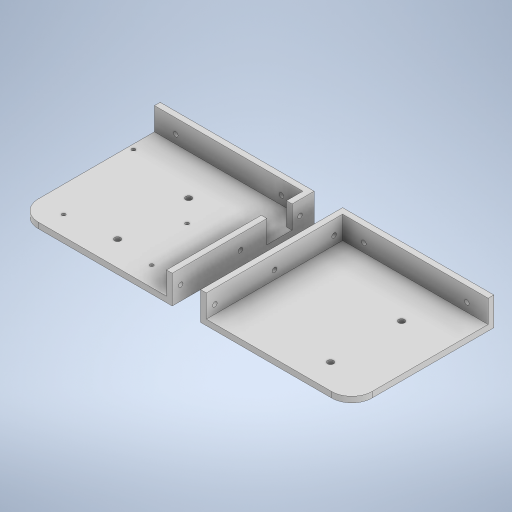
# Autodesk Inventor part: electronics mount
Saved by Autodesk Inventor 2023.1 (Build 271208000, 208)
## iProperties
Created: 2022-11-03
Part Number: electronics mount
Material: Generic
Document SubType Name: Modeling
Designer: nicol
Density: 1 g/cm^3
Appearance: Default
Author: nicol
Autodesk Inventor part; units mm, degrees
ref_plane "YZ Plane" through (0, 0, 0) normal (1, 0, 0) x (0, 1, 0)
ref_plane "XZ Plane" through (0, 0, 0) normal (0, 1, 0) x (-1, 0, 0)
ref_plane "XY Plane" through (0, 0, 0) normal (0, 0, 1) x (1, 0, 0)
sketch "Sketch1" plane through (0, 0, 0) normal (0, 1, 0) x (-1, 0, 0)
  line L0 (108.5, -115) -> (0, -115) construction
  line L1 (0, -115) -> (0, 169.9168) construction
  line L2 (88.5, 0) -> (-126.5, 0) construction
  line L3 (-126.5, 0) -> (-126.5, -115) construction
  line L4 (-126.5, -115) -> (88.5, -115) construction
  line L5 (88.5, -115) -> (88.5, 0) construction
  line L6 (108.5, -15) -> (0, -15)
  line L7 (0, -15) -> (0, -115)
  line L8 (0, -115) -> (108.5, -115)
  line L9 (108.5, -115) -> (108.5, -15)
  line L10 (-20, 169.9168) -> (-20, -115) construction
  line L11 (-20, -15) -> (-126.5, -15)
  line L12 (-126.5, -15) -> (-126.5, -115)
  line L13 (-126.5, -115) -> (-20, -115)
  line L14 (-20, -115) -> (-20, -15)
  point P0 (0, 0)
  point P1 (56, -32.5)
  point P2 (56, -82.5)
  point P3 (-94, -32.5)
  point P4 (-94, -82.5)
  dimension "d4" = 108.5
  dimension "d5" = 20
  dimension "d6" = 215
  dimension "d7" = 115
  dimension "d8" = 20
  dimension "d9" = 50
  dimension "d10" = 150
  dimension "d11" = 32.5
  dimension "d12" = 32.5
  dimension "d13" = 15
  constraints: 30 end point, 7 collinear, 6 parallel, 4 horizontal, 4 perpendicular, 3 point on line, 2 horizontal alignment, 2 vertical alignment, 1 vertical
  measures "d4" distance of L0.start L0.end
  measures "d5" distance between parallel lines of L10 L1
  measures "d6" distance of L2.start L2.end
  measures "d7" distance of L4.end L2.start
  measures "d8" distance of L0.start L4.end
  measures "d9" distance of point (56, -32.5) point (56, -82.5)
  measures "d10" distance of point (-94, -82.5) point (56, -82.5)
  measures "d11" distance from line of L2 point (-94, -32.5)
  measures "d12" distance from line of L5 point (56, -32.5)
  measures "d13" distance between parallel lines of L2 L6
extrude "Extrusion1" add sketch "Sketch1" against normal blind 4
hole "Hole1" at (-56, 0, -32.5) at (-56, 0, -82.5) at (94, 0, -32.5) at (94, 0, -82.5) direction (0, -1, 0) diameter 4.2 end through all
sketch "Sketch2" plane through (0, 0, 0) normal (0, 1, 0) x (1, 0, 0)
  circle A0 centre (-56, 32.5) radius 2.1 projected
  circle A1 centre (-56, 82.5) radius 2.1 projected
  line L0 (0, 15) -> (0, 115) projected
  line L1 (0, 115) -> (-108.5, 115) projected
  line L2 (-108.5, 115) -> (-108.5, 15) projected
  line L3 (-108.5, 15) -> (0, 15) projected
  line L4 (-108.5, 111) -> (-4, 111)
  line L5 (-4, 111) -> (-4, 15)
  line L6 (-108.5, 15) -> (0, 15) projected
  line L7 (0, 115) -> (-108.5, 115) projected
  line L8 (0, 15) -> (0, 115) projected
  circle A2 centre (94, 32.5) radius 2.1 projected
  circle A3 centre (94, 82.5) radius 2.1 projected
  line L9 (126.5, 15) -> (126.5, 115) projected
  line L10 (126.5, 115) -> (20, 115) projected
  line L11 (20, 115) -> (20, 15) projected
  line L12 (20, 15) -> (126.5, 15) projected
  line L13 (126.5, 15) -> (20, 15) projected
  line L14 (24, 15) -> (24, 111)
  line L15 (24, 111) -> (126.5, 111)
  line L16 (20, 115) -> (20, 15) projected
  point P0 (0, 0)
  dimension "d23" = 4
  dimension "d24" = 4
  dimension "d27" = 4
  dimension "d28" = 4
  constraints: 8 end point, 4 parallel, 4 point on line, 2 vertical
  measures "d23" distance between parallel lines of L1 L4
  measures "d24" distance between parallel lines of L0 L5
  measures "d27" distance between parallel lines of L11 L14
  measures "d28" distance between parallel lines of L10 L15
extrude "Extrusion2" add sketch "Sketch2" along normal blind 16 contours L3 L5 L4 L2 L1 L0 | L15 L14 L12 L11 L10 L9
sketch "Sketch3" plane through (0, 0, 0) normal (0, 1, 0) x (1, 0, 0)
  circle A0 centre (-28.1438, 28.659) radius 1.6 projected
  circle A1 centre (-10.1763, 63.5709) radius 1.6 projected
  circle A2 centre (-41.1294, 66.5587) radius 1.6 projected
  circle A3 centre (-105.0821, 92.7675) radius 1.6 projected
  circle A4 centre (-90.06, 28.5422) radius 1.6 projected
  point P0 (0, 0)
hole "Hole2" at (-105.0821, 0, -92.7675) at (-90.06, 0, -28.5422) at (-41.1294, 0, -66.5587) at (-10.1763, 0, -63.5709) at (-28.1438, 0, -28.659) direction (0, -1, 0) diameter 2.5 end through all
sketch "Sketch4" plane through (0, 16, 0) normal (0, 1, 0) x (1, 0, 0)
  line L0 (-5.5415, 99.432) -> (2.2657, 99.432)
  line L1 (2.2657, 99.432) -> (2.2657, 81.6963)
  line L2 (2.2657, 81.6963) -> (-5.5415, 81.6963)
  line L3 (-5.5415, 81.6963) -> (-5.5415, 99.432)
  point P0 (0, 0)
  constraints: 8 end point, 2 parallel, 1 horizontal, 1 perpendicular
extrude "Extrusion3" cut sketch "Sketch4" against normal up to surface (16 mm away)
sketch "Sketch5" plane through (-4, 0, -15) normal (-1, 0, 0) x (0, 0, 1)
  line L0 (-66.6963, 16) -> (0, 16) projected
  line L1 (-96, 0) -> (-96, 16) projected
  line L2 (0, 0) -> (0, 16) projected
  point P0 (15, 0)
  point P1 (-6, 6)
  point P2 (-48, 6)
  point P3 (-90, 6)
  dimension "d38" = 42
  dimension "d39" = 42
  dimension "d40" = 10
  dimension "d41" = 6
  dimension "d42" = 6
  constraints: 2 horizontal alignment
  measures "d38" distance of point (-48, 6) point (-90, 6)
  measures "d39" distance of point (-48, 6) point (-6, 6)
  measures "d40" distance from line of L0 point (-6, 6)
  measures "d41" distance from line of L1 point (-90, 6)
  measures "d42" distance from line of L2 point (-6, 6)
hole "Hole3" at (-4, 6, -21) at (-4, 6, -63) at (-4, 6, -105) direction (1, 0, 0) diameter 3.2 end through all
sketch "Sketch6" plane through (-108.5, 0, -111) normal (0, 0, 1) x (1, 0, 0)
  line L0 (104.5, 0) -> (0, 0) projected
  line L1 (104.5, 0) -> (104.5, 16) projected
  line L2 (0, 16) -> (104.5, 16) projected
  line L3 (0, 0) -> (0, 16) projected
  line L4 (235, 0) -> (132.5, 0) projected
  line L5 (235, 0) -> (235, 16) projected
  line L6 (132.5, 16) -> (235, 16) projected
  line L7 (132.5, 0) -> (132.5, 16) projected
  point P0 (108.5, 0)
  point P1 (15, 6)
  point P2 (89.5, 6)
  point P3 (147.5, 6)
  point P4 (220, 6)
  dimension "d50" = 10
  dimension "d51" = 15
  dimension "d52" = 15
  dimension "d53" = 15
  dimension "d54" = 15
  constraints: 3 horizontal alignment
  measures "d50" distance from line of L2 point (15, 6)
  measures "d51" distance from line of L3 point (15, 6)
  measures "d52" distance from line of L1 point (89.5, 6)
  measures "d53" distance from line of L7 point (147.5, 6)
  measures "d54" distance from line of L5 point (220, 6)
hole "Hole4" at (-93.5, 6, -111) at (-19, 6, -111) at (39, 6, -111) at (111.5, 6, -111) direction (0, 0, -1) diameter 3.2 end through all
fillet "Fillet1" radius 14.25 2 edges at (-108.5, -2, -15) (126.5, -2, -15)
equation "\"d24\" = d23"
equation "\"d27\" = d24"
equation "\"d28\" = d27"
equation "\"d39\" = d38"
body "Solid1"
